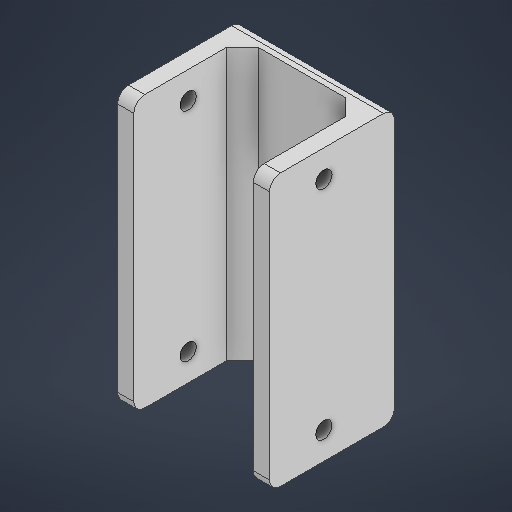
# Autodesk Inventor part: Front_Wheel_Stand
Saved by Autodesk Inventor 2026.1 (Build 301233020, 233B)
## iProperties
Created: 2025-11-03
Part Number: Front_Wheel_Stand
Material: Generic
Document SubType Name: Modeling
Designer: Garfieldcmix
Density: 1 g/cm^3
Appearance: Default
Author: Garfieldcmix
Autodesk Inventor part; units mm, degrees
ref_plane "YZ Plane" through (0, 0, 0) normal (1, 0, 0) x (0, 1, 0)
ref_plane "XZ Plane" through (0, 0, 0) normal (0, 1, 0) x (-1, 0, 0)
ref_plane "XY Plane" through (0, 0, 0) normal (0, 0, 1) x (1, 0, 0)
sketch "Sketch1" plane through (0, 0, 0) normal (0, 1, 0) x (-1, 0, 0)
  line L0 (0, 0) -> (0, -23)
  line L1 (0, -23) -> (-28, -23)
  line L2 (-28, -23) -> (-28, 0)
  line L3 (-28, 0) -> (-25, 0)
  line L4 (-25, 0) -> (-25, -20)
  line L5 (-25, -20) -> (-3, -20)
  line L6 (-3, -20) -> (-3, 0)
  line L7 (-3, 0) -> (0, 0)
  dimension "d0" = 3
  dimension "d1" = 3
  dimension "d2" = 3
  dimension "d3" = 28
  dimension "d4" = 23
  constraints: 16 end point, 7 perpendicular, 1 point on line, 1 vertical
  measures "d0" distance of L6.end L0.start
  measures "d1" distance of L2.end L3.end
  measures "d2" distance between parallel lines of L1 L5
  measures "d3" distance of L0.end L1.end
  measures "d4" distance of L0.start L0.end
extrude "Extrusion1" add sketch "Sketch1" along normal blind 50
sketch "Sketch2" plane through (0, 0, -23) normal (-1, 0, 0) x (0, 0, 1)
  circle A0 centre (13, 45) radius 1.5
  circle A1 centre (13, 5) radius 1.5
  line L0 (23, 0) -> (23, 50) construction
  line L1 (13, 5) -> (13, 45) construction
  line L2 (0, 0) -> (23, 0) construction
  dimension "d8" = 3
  dimension "d9" = 10
  dimension "d11" = 40
  dimension "d12" = 5
  constraints: 2 centre point, 2 end point, 1 equal radius, 1 vertical
  measures "d8" diameter of A1
  measures "d9" distance from line of L0 L1.start
  measures "d11" distance of L1.start L1.end
  measures "d12" distance from line of L2 L1.start
extrude "Extrusion2" cut sketch "Sketch2" against normal up to surface (28 mm away)
fillet "Fillet1" radius 2 6 edges at (1.5, 50, 0) (1.5, 0, 0) (26.5, 50, 0) (26.5, 0, 0) (14, 50, -23) (14, 0, -23)
chamfer "Chamfer1" distance 3 angle 45 2 edges at (3, 25, -20) (25, 25, -20)
body "Solid1"
